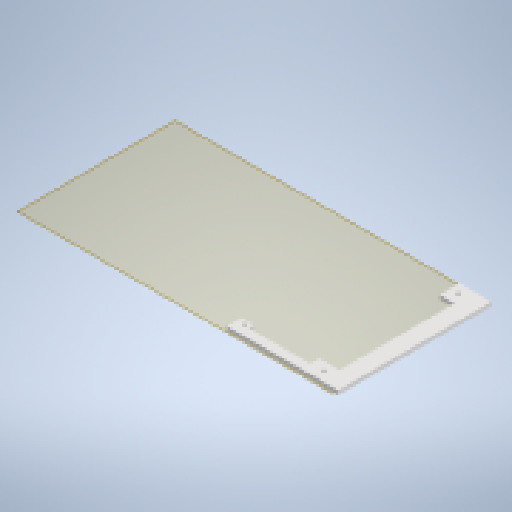
# Autodesk Inventor part: strut1
Saved by Autodesk Inventor 2024 (Build 280153000, 153)
## iProperties
Created: 2024-10-10
Part Number: strut1
Material: Generic
Document SubType Name: Modeling
Designer: PC
Density: 1 g/cm^3
Appearance: Default
Author: PC
Autodesk Inventor part; units mm, degrees
ref_plane "YZ Plane" through (0, 0, 0) normal (1, 0, 0) x (0, 1, 0)
ref_plane "XZ Plane" through (0, 0, 0) normal (0, 1, 0) x (-1, 0, 0)
ref_plane "XY Plane" through (0, 0, 0) normal (0, 0, 1) x (1, 0, 0)
ref_plane "Work Plane1" through (-100.0042, 32.3083, -20.5972) normal (0, 1, 0) x (-1, 0, 0)
sketch "Sketch2" plane through (-100.0042, 32.3083, -20.5972) normal (0, 1, 0) x (-1, 0, 0)
  line L0 (-37.0577, 56.8227) -> (-118.6401, 56.8227)
  line L1 (-118.6401, 56.8227) -> (-118.6401, -55.8539)
  line L2 (-118.6401, -55.8539) -> (-95.0834, -55.8539)
  line L3 (-95.0834, -55.8539) -> (-95.0834, -41.3074)
  line L4 (-95.0834, -41.3074) -> (-106.1561, -41.3074)
  line L5 (-106.1561, -41.3074) -> (-106.1561, 43.3122)
  line L6 (-106.1561, 43.3122) -> (-91.4467, 43.3122)
  line L7 (-105, 46) -> (-105, -52.5) projected
  line L8 (-105, -52.5) -> (105, -52.5) projected
  line L9 (105, -52.5) -> (105, 52.5) projected
  line L10 (105, 52.5) -> (-93, 52.5) projected
  line L11 (-93, 52.5) -> (-93, 48) projected
  arc A0 (-95, 46) -> (-93, 48) centre (-95, 48) ccw projected
  line L12 (-95, 46) -> (-105, 46) projected
  circle A1 centre (-101, -48.5) radius 1.5 projected
  circle A2 centre (101, -48.5) radius 2 projected
  circle A3 centre (101, 27.5) radius 2 projected
  circle A4 centre (-42.4, 49.5) radius 1.5 projected
  circle A5 centre (-101, -48.5) radius 1.5 projected
  circle A6 centre (-101, -48.5) radius 1.5 projected
  circle A7 centre (-101, -48.5) radius 1.5 projected
  circle A8 centre (-101, -48.5) radius 1.5 projected
  circle A9 centre (-101, -48.5) radius 1.5 projected
  circle A10 centre (-101, -48.5) radius 1.5 projected
  circle A11 centre (-101, -48.5) radius 1.5 projected
  circle A12 centre (-101, -48.5) radius 1.5 projected
  circle A13 centre (-101, -48.5) radius 1.5 projected
  circle A14 centre (-101, -48.5) radius 1.45
  circle A15 centre (-101, 49.5) radius 1.45
  line L13 (-91.4467, 50.0155) -> (-46.3722, 50.0155)
  line L14 (-46.3722, 50.0155) -> (-46.3722, 46)
  line L15 (-46.3722, 46) -> (-37.0577, 46)
  line L16 (-37.0577, 46) -> (-37.0577, 56.8227)
  line L17 (-91.4467, 43.3122) -> (-91.4467, 50.0155)
  circle A16 centre (-42.4, 49.5) radius 1.5
  point P0 (-100.0042, 20.5972)
  point P1 (-37.0577, 56.8227)
  dimension "d2" = 2.9
  constraints: 24 end point, 9 perpendicular, 3 centre point, 3 coincident, 2 horizontal, 2 vertical, 1 concentric, 2 other
  measures "d2" diameter of A14
extrude "Extrusion1" add sketch "Sketch2" along normal blind 3 contours L16 L10 L11 A0 L12 L7 L6 L5 L4 L8 L3 L2 L1 L0 | L16 L15 L14 L13 L17 L6 L7 L12 A0 L11 L10 | L8 L7 L4 L3
body "Solid1"
